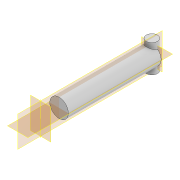
# Autodesk Inventor part: UpperlegP
Saved by Autodesk Inventor 2021 (Build 250183000, 183)
## iProperties
Created: 2020-12-19
Part Number: UpperlegP
Material: 一般
Document SubType Name: Modeling
Designer: Tazaki
Density: 2.84589 g/cm^3
Appearance: 既定
Mass: 1500 g
Surface Area: 474.022 cm^2
Volume: 527.076 cm^3
Author: Tazaki
Autodesk Inventor part; units mm, degrees
ref_plane "作業平面1" through (0, 0, -300) normal (0, 0, 1) x (1, 0, 0)
sketch "スケッチ3" plane through (0, 0, 0) normal (0, 0, 1) x (1, 0, 0)
  circle A0 centre (0, 0) radius 25
  dimension "d7" = 50
  constraints: 1 centre point, 1 coincident
  measures "d7" diameter of A0
extrude "押し出し2" add sketch "スケッチ3" against normal blind 300
sketch "スケッチ4" plane through (0, 0, 0) normal (1, 0, 0) x (0, 1, 0)
  line L0 (82.0674, 98.3645) -> (-82.6495, 98.3645)
  line L1 (-82.6495, 98.3645) -> (-82.6495, -50)
  line L2 (-82.6495, -50) -> (82.0674, -50)
  line L3 (82.0674, -50) -> (82.0674, 98.3645)
  line L4 (-115.5929, 0) -> (115.0108, 0) projected
  point P0 (0, 0)
  dimension "d10" = 50
  constraints: 8 end point, 2 parallel, 1 horizontal, 1 perpendicular
  measures "d10" distance between parallel lines of L2 L4
extrude "押し出し3" cut sketch "スケッチ4" along normal mid plane 300
sketch "スケッチ5" plane through (0, 0, 0) normal (0, 1, 0) x (-1, 0, 0)
  circle A0 centre (0, -300) radius 15
  point P0 (0, 0)
  dimension "d13" = 30
  dimension "d14" = 300
  constraints: 1 centre point, 1 vertical alignment
  measures "d13" diameter of A0
  measures "d14" distance of point (0, 0) A0.centre
extrude "押し出し4" add sketch "スケッチ5" along normal mid plane 75
